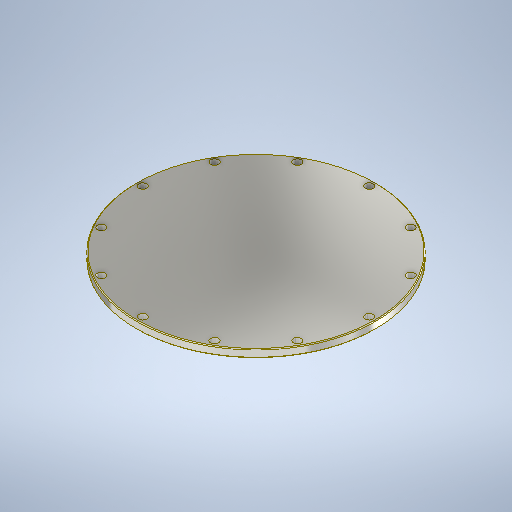
# Autodesk Inventor part: 101 part 1
Saved by Autodesk Inventor 2025.1 (Build 291241000, 241)
## iProperties
Created: 2024-09-02
Part Number: 101 part 1
Material: Silver
Document SubType Name: Modeling
Designer: ffogue
Density: 10.49 g/cm^3
Appearance: Silver
Author: ffogue
Autodesk Inventor part; units mm, degrees
ref_plane "YZ Plane" through (0, 0, 0) normal (1, 0, 0) x (0, 1, 0)
ref_plane "XZ Plane" through (0, 0, 0) normal (0, 1, 0) x (-1, 0, 0)
ref_plane "XY Plane" through (0, 0, 0) normal (0, 0, 1) x (1, 0, 0)
sketch "Sketch1" plane through (0, 0, 0) normal (0, 0, 1) x (1, 0, 0)
  circle A0 centre (0, 0) radius 75.5
  dimension "d0" = 151
  constraints: 1 centre point, 1 coincident
  measures "d0" diameter of A0
extrude "Extrusion1" add sketch "Sketch1" against normal blind 5
sketch "Sketch2" plane through (0, 0, 0) normal (0, 0, 1) x (1, 0, 0)
  circle A0 centre (0, 0) radius 71.5 construction
  point P0 (0, 71.5)
  dimension "d3" = 143
  constraints: 2 vertical alignment, 1 coincident, 2 other
hole "Hole1" at (0, 71.5, 0) direction (0, 0, -1) diameter 5 depth 5
pattern_circular "Circular Pattern1" count 12 over 360 about axis through (0, 0, 0) along (0, 0, -1) of "Hole1"
fillet "Fillet1" radius 0.5 2 edges at (-75.5, 0, 0) (-75.5, 0, -5)
body "Solid1"
